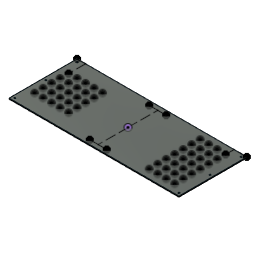
240x600mm Plate v32 (Autodesk Fusion 360 design; units mm, degrees)
Autodesk Fusion 360 part; units mm, degrees
sketch "Main" plane through (0, 0, 0) normal (0, 0, 1) x (1, 0, 0)
  line L0 (300, 120) -> (-300, 120)
  line L1 (-300, 120) -> (-300, -120)
  line L2 (-300, -120) -> (300, -120)
  line L3 (300, -120) -> (300, 120)
  line L4 (300, 120) -> (-300, -120) construction
  line L5 (-300, 120) -> (300, -120) construction
  line L6 (-300, 120) -> (-290, 120) construction
  line L7 (-290, 120) -> (-290, 110) construction
  circle A0 centre (-290, 110) radius 2.75
  circle A1 centre (290, 110) radius 2.75
  circle A2 centre (-290, 0) radius 2.75
  circle A3 centre (290, 0) radius 2.75
  circle A4 centre (-290, -110) radius 2.75
  circle A5 centre (290, -110) radius 2.75
  dimension "d5" = 600
  dimension "d6" = 240
  dimension "d8" = 10
  dimension "d9" = 10
  dimension "d10" = 5.5
  dimension "d13" = 580
  dimension "d14" = -220
  constraint horizontal L0
  constraint perpendicular L0 L1
  constraint parallel L0 L2
  constraint parallel L1 L3
  constraint coincident L4 origin
  constraint coincident L5 origin
  constraint perpendicular L1 L6
  constraint vertical L7
  constraint coincident L7.end A0.centre
  measures "d5" distance of L1.end L2.end
  measures "d6" distance of L0.end L1.end
  measures "d8" distance of L0.end L6.end
  measures "d9" distance of L6.end L7.end
  measures "d10" diameter of A0
extrude "Extrude1" add sketch "Main" along normal blind 3
sketch "Tool holes" plane through (0, 0, 3) normal (0, 0, 1) x (-1, 0, 0)
  circle A0 centre (-290, 110) radius 2.75
  circle A1 centre (290, 110) radius 2.75
  circle A2 centre (-290, -110) radius 2.75
  circle A3 centre (290, 0) radius 2.75
  circle A4 centre (-290, 0) radius 2.75
  circle A5 centre (290, -110) radius 2.75
  line L0 (-300, 120) -> (-300, -120)
  line L1 (-300, -120) -> (300, -120)
  line L2 (300, -120) -> (300, 120)
  line L3 (300, 120) -> (-300, 120)
  line L4 (300, -120) -> (270, -120) construction
  line L5 (270, -120) -> (270, -60) construction
  circle A6 centre (270, -60) radius 1.5
  circle A7 centre (240, -60) radius 1.5
  circle A8 centre (210, -60) radius 1.5
  circle A9 centre (270, -30) radius 1.5
  circle A10 centre (240, -30) radius 1.5
  circle A11 centre (210, -30) radius 1.5
  circle A12 centre (270, 0) radius 1.5
  circle A13 centre (240, 0) radius 1.5
  circle A14 centre (210, 0) radius 1.5
  circle A15 centre (270, 30) radius 1.5
  circle A16 centre (240, 30) radius 1.5
  circle A17 centre (210, 30) radius 1.5
  circle A18 centre (270, 60) radius 1.5
  circle A19 centre (240, 60) radius 1.5
  circle A20 centre (210, 60) radius 1.5
  circle A21 centre (180, -60) radius 1.5
  circle A22 centre (150, -60) radius 1.5
  circle A23 centre (180, -30) radius 1.5
  circle A24 centre (150, -30) radius 1.5
  circle A25 centre (180, 0) radius 1.5
  circle A26 centre (150, 0) radius 1.5
  circle A27 centre (180, 30) radius 1.5
  circle A28 centre (150, 30) radius 1.5
  circle A29 centre (180, 60) radius 1.5
  circle A30 centre (150, 60) radius 1.5
  line L6 (-300, -120) -> (-255, -120) construction
  line L7 (-255, -120) -> (-255, -90) construction
  circle A31 centre (-255, -90) radius 1.5
  circle A32 centre (-225, -90) radius 1.5
  circle A33 centre (-195, -90) radius 1.5
  circle A34 centre (-255, -60) radius 1.5
  circle A35 centre (-225, -60) radius 1.5
  circle A36 centre (-195, -60) radius 1.5
  circle A37 centre (-255, -30) radius 1.5
  circle A38 centre (-225, -30) radius 1.5
  circle A39 centre (-195, -30) radius 1.5
  circle A40 centre (-165, -90) radius 1.5
  circle A41 centre (-165, -60) radius 1.5
  circle A42 centre (-165, -30) radius 1.5
  circle A43 centre (-255, 0) radius 1.5
  circle A44 centre (-225, 0) radius 1.5
  circle A45 centre (-195, 0) radius 1.5
  circle A46 centre (-165, 0) radius 1.5
  circle A47 centre (-255, 30) radius 1.5
  circle A48 centre (-225, 30) radius 1.5
  circle A49 centre (-195, 30) radius 1.5
  circle A50 centre (-165, 30) radius 1.5
  circle A51 centre (-255, 60) radius 1.5
  circle A52 centre (-225, 60) radius 1.5
  circle A53 centre (-195, 60) radius 1.5
  circle A54 centre (-165, 60) radius 1.5
  circle A55 centre (-255, 90) radius 1.5
  circle A56 centre (-225, 90) radius 1.5
  circle A57 centre (-195, 90) radius 1.5
  circle A58 centre (-165, 90) radius 1.5
  line L8 (0, 0) -> (0, -105) construction
  line L9 (0, -105) -> (-30, -105) construction
  line L10 (0, -105) -> (30, -105) construction
  circle A59 centre (30, -105) radius 1.5
  circle A60 centre (-30, -105) radius 1.5
  line L11 (0, 0) -> (0, 105) construction
  line L12 (0, 105) -> (-30, 105) construction
  line L13 (0, 105) -> (30, 105) construction
  circle A61 centre (30, 105) radius 1.5
  circle A62 centre (-30, 105) radius 1.5
  dimension "d21" = 30
  dimension "d22" = 60
  dimension "d23" = 3
  dimension "d26" = -120
  dimension "d27" = 120
  dimension "d36" = 45
  dimension "d37" = 30
  dimension "d38" = 3
  dimension "d41" = 90
  dimension "d42" = 180
  dimension "d50" = 105
  dimension "d51" = 30
  dimension "d52" = 30
  dimension "d53" = 3
  dimension "d54" = 3
  dimension "d55" = 105
  dimension "d56" = 30
  dimension "d57" = 30
  dimension "d58" = 3
  dimension "d59" = 3
  constraint coincident L1.end L2.start
  constraint perpendicular L2 L4
  constraint perpendicular L1 L5
  constraint coincident L5.end A6.centre
  constraint coincident L0.end L1.start
  constraint perpendicular L0 L6
  constraint perpendicular L1 L7
  constraint coincident L7.end A31.centre
  constraint coincident L8.start L11.start
  constraint vertical L8
  constraint perpendicular L8 L9
  constraint perpendicular L8 L10
  constraint coincident L10.end A59.centre
  constraint coincident L9.end A60.centre
  constraint parallel L8 L11
  constraint perpendicular L11 L12
  constraint perpendicular L11 L13
  constraint coincident L13.end A61.centre
  constraint coincident L12.end A62.centre
  measures "d21" distance of L1.end L4.end
  measures "d22" distance of L4.end L5.end
  measures "d23" diameter of A6
  measures "d36" distance of L0.end L6.end
  measures "d37" distance of L6.end L7.end
  measures "d38" diameter of A31
  measures "d50" distance of L8.start L8.end
  measures "d51" distance of L8.end L9.end
  measures "d52" distance of L8.end L10.end
  measures "d53" diameter of A59
  measures "d54" diameter of A60
  measures "d55" distance of L8.start L11.end
  measures "d56" distance of L11.end L12.end
  measures "d57" distance of L11.end L13.end
  measures "d58" diameter of A61
  measures "d59" diameter of A62
extrude "Extrude2" cut sketch "Tool holes" against normal blind 3 contours A6 | A7 | A8 | A9 | A10 | A11 | A12 | A13 | A14 | A15 | A16 | A17 | A18 | A19 | A20 | A21 | A22 | A23 | A24 | A25 | A26 | A27 | A28 | A29 | A30
extrude "Extrude3" cut sketch "Tool holes" against normal blind 3 contours A6 | A7 | A8 | A9 | A10 | A11 | A12 | A13 | A14 | A15 | A16 | A17 | A18 | A19 | A20 | A21 | A22 | A23 | A24 | A25 | A26 | A27 | A28 | A29 | A30 | A31 | A32 | A33 | A34 | A35 | A36 | A37 | A38 | A39 | A40 | A41 | A42 | A43 | A44 | A45 | A46 | A47 | A48 | A49 | A50 | A51 | A52 | A53 | A54 | A55 | A56 | A57 | A58 | A59 | A60 | A61 | A62
equation "x = 600 mm"
equation "y = 240 mm"
equation "mounting_hole_d = 5.5 mm"
equation "tool_hole_d = 3 mm"
equation "d5 = x"
equation "d6 = y"
equation "mounting_hole_dist_from_side = 10 mm"
equation "d8 = mounting_hole_dist_from_side"
equation "d9 = mounting_hole_dist_from_side"
equation "d10 = mounting_hole_d"
equation "d13 = x - 2 * mounting_hole_dist_from_side"
equation "d14 = -1 * ( y - 2 * mounting_hole_dist_from_side )"
equation "z = 3 mm" comment "material thickness"
equation "d16 = z"
equation "d21 = tool_holes_x_side_offset"
equation "d22 = tool_holes_y_side_offset"
equation "d23 = tool_hole_d"
equation "d24 = tool_holes_x_amount"
equation "d25 = tool_holes_y_amount"
equation "d26 = ( -1 + tool_holes_x_amount ) * tool_holes_spacing * -1"
equation "d27 = y - ( 2 * tool_holes_y_side_offset )"
equation "tool_holes_spacing = 30 mm"
equation "tool_holes_y_side_offset = 60 mm"
equation "tool_holes_x_side_offset = 30 mm"
equation "tool_holes_x_amount = 5"
equation "d33 = -z"
equation "tool_holes_x_side_offset2 = 45 mm"
equation "d36 = tool_holes_x_side_offset2"
equation "d37 = tool_holes_y_side_offset2"
equation "d38 = tool_hole_d"
equation "d39 = tool_holes_x_amount2"
equation "d40 = tool_holes_y_amount2"
equation "d41 = ( -1 + tool_holes_x_amount2 ) * tool_holes_spacing"
equation "d42 = y - ( 2 * tool_holes_y_side_offset2 )"
equation "tool_holes_y_amount = 5" comment "isnt correctly parameterized, when changed"
equation "tool_holes_y_side_offset2 = 30 mm"
equation "tool_holes_y_amount2 = 7"
equation "tool_holes_x_amount2 = 4"
equation "support_foot_hole_spacing = 60 mm"
equation "support_foot_side_offset = 15 mm"
equation "d50 = y / 2 - support_foot_side_offset"
equation "d51 = support_foot_hole_spacing * 0.5"
equation "d52 = support_foot_hole_spacing * 0.5"
equation "d53 = tool_hole_d"
equation "d54 = tool_hole_d"
equation "d55 = y / 2 - support_foot_side_offset"
equation "d56 = support_foot_hole_spacing * 0.5"
equation "d57 = support_foot_hole_spacing * 0.5"
equation "d58 = tool_hole_d"
equation "d59 = tool_hole_d"
equation "d60 = -z"
